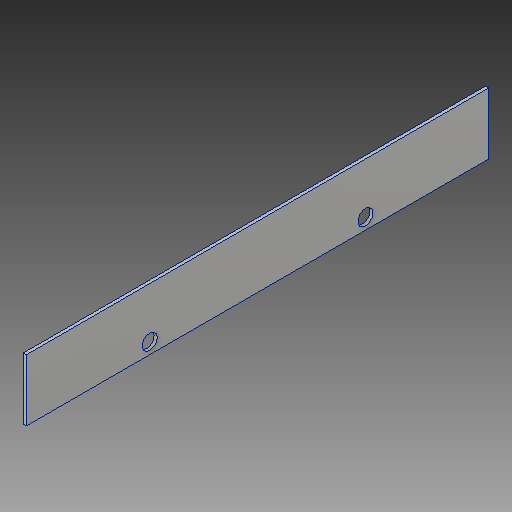
# Autodesk Inventor part: Bumper Plate
Saved by Autodesk Inventor 2019 (Build 230136000, 136)
## iProperties
Created: 2019-11-03
Part Number: Bumper Plate
Material: Aluminum 6061
Document SubType Name: Modeling
Designer: admin
Density: 2.7 g/cm^3
Appearance: Aluminum - Flat
Author: admin
Autodesk Inventor part; units mm, degrees
ref_plane "YZ Plane" through (0, 0, 0) normal (1, 0, 0) x (0, 1, 0)
ref_plane "XZ Plane" through (0, 0, 0) normal (0, 1, 0) x (-1, 0, 0)
ref_plane "XY Plane" through (0, 0, 0) normal (0, 0, 1) x (1, 0, 0)
sketch "Sketch1" plane through (0, 0, 0) normal (1, 0, 0) x (0, 1, 0)
  line L0 (-50, 375) -> (50, 375)
  line L1 (50, 375) -> (50, -375)
  line L2 (50, -375) -> (-50, -375)
  line L3 (-50, -375) -> (-50, 375)
  line L4 (-50, 375) -> (50, -375) construction
  line L5 (50, 375) -> (-50, -375) construction
  point P0 (0, 0)
  dimension "d0" = 100
  dimension "d1" = 750
  constraints: 12 end point, 2 midpoint, 2 parallel, 1 horizontal, 1 perpendicular
  measures "d0" distance of L1.end L2.end
  measures "d1" distance of L0.end L1.end
extrude "Extrusion1" add sketch "Sketch1" along normal blind 5
sketch "Sketch2" plane through (5, 0, 0) normal (1, 0, 0) x (0, 0, -1)
  circle A0 centre (-175, -31.7) radius 12.3
  line L0 (-375, -50) -> (375, -50) projected
  line L1 (-375, 50) -> (-375, -50) projected
  line L2 (375, 50) -> (-375, 50) projected
  line L3 (0, 50) -> (0, -50)
  circle A1 centre (175, -31.7) radius 12.3
  point P0 (0, 0)
  dimension "d4" = 18.3
  dimension "d5" = 200
  dimension "d6" = 24.6
  dimension "d9" = 375
  constraints: 2 centre point, 2 end point, 2 midpoint, 1 perpendicular, 1 symmetric about line, 1 other
  measures "d4" distance from line of L0 A0.centre
  measures "d5" distance from line of L1 A0.centre
  measures "d6" diameter of A0
  measures "d9" distance between parallel lines of L1 L3
extrude "Extrusion2" cut sketch "Sketch2" against normal through all contours A0 | A1
body "Solid1"
